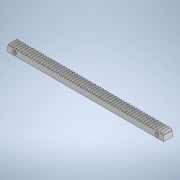
# Autodesk Inventor part: Rack
Saved by Autodesk Inventor 2022 (Build 260153000, 153)
## iProperties
Created: 2022-08-19
Part Number: Rack
Material: Generico
Document SubType Name: Modeling
Designer: matte
Density: 1 g/cm^3
Appearance: Default
Author: matte
Autodesk Inventor part; units mm, degrees
ref_plane "YZ Plane" through (0, 0, 0) normal (1, 0, 0) x (0, 1, 0)
ref_plane "XZ Plane" through (0, 0, 0) normal (0, 1, 0) x (-1, 0, 0)
ref_plane "XY Plane" through (0, 0, 0) normal (0, 0, 1) x (1, 0, 0)
sketch "Rettangolo base" plane through (0, 0, 0) normal (0, 0, 1) x (1, 0, 0)
  line L0 (-141.3717, 5) -> (141.3717, 5)
  line L1 (141.3717, 5) -> (141.3717, -5)
  line L2 (141.3717, -5) -> (-141.3717, -5)
  line L3 (-141.3717, -5) -> (-141.3717, 5)
  point P0 (0, 0)
  point P1 (0, 5)
  point P2 (141.3717, 0)
  dimension "d0" = 282.7433
  dimension "d1" = 10
  constraints: 8 end point, 2 midpoint, 2 parallel, 1 horizontal, 1 horizontal alignment, 1 perpendicular, 1 vertical alignment
  measures "d0" distance of L1.end L2.end
  measures "d1" distance between parallel lines of L0 L2
extrude "Estrusione1" add sketch "Rettangolo base" along normal blind 15.5
sketch "Trapezio dente" plane through (0, 0, 15.5) normal (0, 0, 1) x (1, 0, 0)
  line L0 (-140.876, 5) -> (-139.6476, 8.375)
  line L1 (-139.6476, 8.375) -> (-138.3833, 8.375)
  line L2 (-138.3833, 8.375) -> (-137.1549, 5)
  line L3 (-139.0155, 38.945) -> (-139.0155, 10.1058) construction
  line L4 (141.3717, 5) -> (-141.3717, 5) construction
  line L5 (-140.1936, 6.875) -> (-137.8374, 6.875) construction
  line L6 (-140.876, 5) -> (-137.1549, 5)
  line L7 (-141.3717, 5) -> (-141.3717, -5) projected
  point P0 (0, 0)
  dimension "d4" = 40
  dimension "d6" = 1.5
  dimension "d7" = 2.3562
  dimension "d15" = 2.3562
  dimension "d25" = 1.875
  constraints: 12 end point, 4 point on line, 2 horizontal, 1 parallel, 1 vertical, 1 other
  measures "d4" angle of L2 L0
  measures "d6" distance between parallel lines of L1 L5
  measures "d7" distance of L5.start L5.end
  measures "d15" distance between parallel lines of L7 L3
  measures "d25" distance between parallel lines of L5 L4
extrude "Estrusione2" add sketch "Trapezio dente" against normal blind 15
fillet "Raccordo1" radius 0.6 1 edges at (-137.1549, 5, 8)
fillet "Raccordo1" radius 0.6 1 edges at (-140.876, 5, 8)
pattern_linear "Serie rettangolare1" count 60 spacing 4.7124 along (1, 0, 0) of "Estrusione2", "Raccordo1"
sketch "Schizzo fori" plane through (0, 0, 15.5) normal (0, 0, 1) x (1, 0, 0)
  line L0 (-141.3717, 5) -> (-141.3717, -5) projected
  line L1 (141.3717, -5) -> (141.3717, 5) projected
  point P0 (0, 0)
  point P1 (-129.3717, 0)
  point P2 (129.3717, 0)
  dimension "d16" = 12
  dimension "d17" = 12
  constraints: 2 horizontal alignment
  measures "d16" distance from line of L0 point (-129.372, 0)
  measures "d17" distance from line of L1 point (129.372, 0)
hole "Foro1" at (-129.3717, 0, 15.5) at (129.3717, 0, 15.5) direction (0, 0, -1) diameter 7 end through all
equation "\"d2\" = spessore_body"
equation "\"d7\" = 1.5708 * m_val"
equation "\"d15\" = 1.5708 * m_val"
equation "\"d8\" = spessore_dente"
equation "\"d14\" = 3.14159 * m_val"
equation "\"d17\" = d16"
equation "\"spessore_dente\" = 15"
equation "\"spessore_body\" = 15.5"
equation "\"m_val\" = 1.5"
equation "\"r_racc\" = 0.6"
